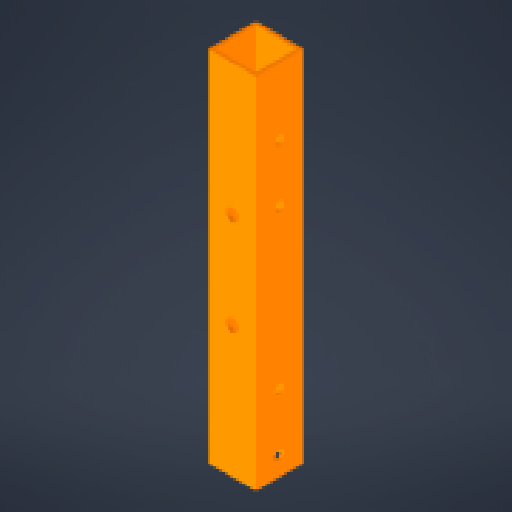
# Autodesk Inventor part: side_axis
Saved by Autodesk Inventor 2024 (Build 280153000, 153)
## iProperties
Created: 2023-10-12
Part Number: side_axis
Material: Типовые
Document SubType Name: Modeling
Designer: user
Density: 1 g/cm^3
Appearance: По умолчанию
Mass: 21.9067 g
Surface Area: 296.853 cm^2
Volume: 21.9067 cm^3
Author: user
Autodesk Inventor part; units mm, degrees
ref_plane "YZ Plane" through (0, 0, 0) normal (1, 0, 0) x (0, 1, 0)
ref_plane "XZ Plane" through (0, 0, 0) normal (0, 1, 0) x (-1, 0, 0)
ref_plane "XY Plane" through (0, 0, 0) normal (0, 0, 1) x (1, 0, 0)
sketch "Эскиз1" plane through (0, 0, 0) normal (0, 0, 1) x (1, 0, 0)
  line L0 (0, 0) -> (17, 0)
  line L1 (17, 0) -> (17, 17)
  line L2 (17, 17) -> (0, 17)
  line L3 (0, 17) -> (0, 0)
  line L4 (-1.5, 18.5) -> (18.5, 18.5)
  line L5 (18.5, 18.5) -> (18.5, -1.5)
  line L6 (18.5, -1.5) -> (-1.5, -1.5)
  line L7 (-1.5, -1.5) -> (-1.5, 18.5)
  dimension "d0" = 20
  dimension "d1" = 1.5
  constraints: 16 end point, 4 parallel, 3 perpendicular, 1 horizontal, 3 other
  measures "d0" distance of L4.start L4.end
  measures "d1" horizontal distance of L4.end L1.end
extrude "Выдавливание1" add sketch "Эскиз1" along normal blind 130
sketch "Эскиз2" plane through (-1.5, 18.5, 0) normal (0, 1, 0) x (1, 0, 0)
  line L0 (20, -130) -> (0, -130) construction
  line L1 (20, 0) -> (0, 0) construction
  line L2 (20, 0) -> (20, -130) construction
  circle A0 centre (10, -52.5) radius 2.75
  circle A1 centre (10, -77.5) radius 2.75
  line L3 (10, -77.5) -> (10, -52.5) construction
  point P0 (1.5, 0)
  point P1 (10, -65)
  point P2 (20, -65)
  point P3 (10, 0)
  dimension "d4" = 25
  dimension "d5" = 5.5
  constraints: 3 midpoint, 2 centre point, 2 end point, 1 equal radius, 1 horizontal alignment, 1 vertical, 1 vertical alignment
  measures "d4" distance of L3.start L3.end
  measures "d5" diameter of A0
extrude "Выдавливание2" cut sketch "Эскиз2" against normal through all
sketch "Эскиз3" plane through (-1.5, -1.5, 0) normal (-1, 0, 0) x (0, 0, 1)
  circle A0 centre (8, 10) radius 2 projected
  circle A1 centre (32, 10) radius 2 projected
  circle A2 centre (98, 10) radius 2 projected
  circle A3 centre (122, 10) radius 2 projected
  point P0 (0, 1.5)
extrude "Выдавливание3" cut sketch "Эскиз3" against normal blind 200
